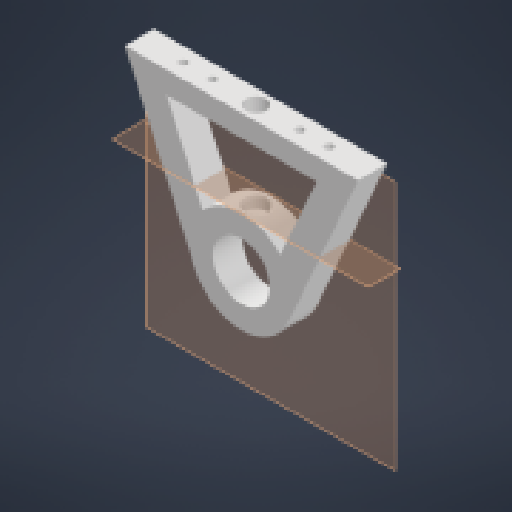
# Autodesk Inventor part: LowerWheelBracket
Saved by Autodesk Inventor 2023 (Build 270158000, 158)
## iProperties
Created: 2023-02-25
Part Number: LowerWheelBracket
Material: Generic
Document SubType Name: Modeling
Designer: izack
Density: 1 g/cm^3
Appearance: Default
Author: izack
Autodesk Inventor part; units mm, degrees
ref_plane "YZ Plane" through (0, 0, 0) normal (1, 0, 0) x (0, 1, 0)
ref_plane "XZ Plane" through (0, 0, 0) normal (0, 1, 0) x (-1, 0, 0)
ref_plane "XY Plane" through (0, 0, 0) normal (0, 0, 1) x (1, 0, 0)
ref_plane "Work Plane1" through (0, 0, 2.5) normal (0, 0, 1) x (1, 0, 0)
sketch "Sketch1" plane through (0, 0, 2.5) normal (0, 0, 1) x (1, 0, 0)
  circle A0 centre (0, 0) radius 9.75
  circle A1 centre (0, 0) radius 17.5
  line L0 (0, 0) -> (0, 47) construction
  line L1 (40, 47) -> (-40, 47)
  line L2 (-40, 47) -> (-15.996, -7.0977)
  line L3 (40, 47) -> (15.996, -7.0977)
  line L4 (-25.7319, 39.5) -> (25.7319, 39.5)
  line L5 (25.7319, 39.5) -> (13.2683, 11.4107)
  line L6 (-13.2683, 11.4107) -> (-25.7319, 39.5)
  dimension "d0" = 19.5
  dimension "d1" = 35
  dimension "d2" = 47
  dimension "d3" = 80
  dimension "d4" = 7.5
  dimension "d6" = 10
  dimension "d7" = 10
  constraints: 14 end point, 4 point on circle, 2 centre point, 2 coincident, 2 horizontal, 2 parallel, 2 tangent, 1 midpoint, 1 vertical
  measures "d0" diameter of A0
  measures "d1" diameter of A1
  measures "d2" distance of L0.start L0.end
  measures "d3" distance of L1.start L1.end
  measures "d4" distance between parallel lines of L4 L1
  measures "d6" distance between parallel lines of L2 L6
  measures "d7" distance between parallel lines of L3 L5
extrude "Extrusion1" add sketch "Sketch1" along normal blind 10 contours A1 | A1 L5 L4 L6 L2 L1 L3
sketch "Sketch2" plane through (-40, 47, 2.5) normal (0, 1, 0) x (1, 0, 0)
  line L0 (0, 0) -> (0, -10) construction
  line L1 (0, -5) -> (80, -5) construction
  line L2 (80, 0) -> (80, -10) construction
  circle A0 centre (15, -5) radius 1.35
  circle A1 centre (25, -5) radius 1.35
  line L3 (40, -5) -> (40, 0) construction
  line L4 (24.004, 0) -> (55.996, 0) construction
  circle A2 centre (65, -5) radius 1.35
  circle A3 centre (55, -5) radius 1.35
  circle A4 centre (40, -5) radius 3.5
  point P0 (40, 2.5)
  dimension "d10" = 2.7
  dimension "d11" = 15
  dimension "d14" = 10
  dimension "d19" = 7
  constraints: 5 centre point, 4 end point, 4 midpoint, 2 symmetric about line, 1 coincident, 1 horizontal, 1 point on line, 4 other
  measures "d10" diameter of A0
  measures "d11" distance from line of L0 A0.centre
  measures "d14" distance of A0.centre A1.centre
  measures "d19" diameter of A4
extrude "Extrusion2" cut sketch "Sketch2" against normal up to surface (7.5 mm away)
ref_plane "Work Plane2" through (-40, 17.5, 2.5) normal (0, 1, 0) x (1, 0, 0)
sketch "Sketch3" plane through (-40, 17.5, 2.5) normal (0, 1, 0) x (1, 0, 0)
  circle A0 centre (40, -5) radius 3.5 projected
  point P0 (40, 2.5)
extrude "Extrusion3" cut sketch "Sketch3" against normal blind 4
fillet "Fillet1" radius 1 3 edges at (2.669, 17.2953, 9.7641) (-3.4999, 17.1465, 7.4721) (2.6638, 17.2961, 5.2297)
body "Solid1"
